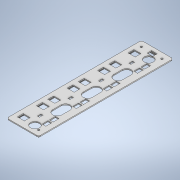
# Autodesk Inventor part: BoxLid
Saved by Autodesk Inventor 2021 (Build 250183000, 183)
## iProperties
Created: 2023-03-09
Part Number: BoxLid
Material: Generic
Document SubType Name: Modeling
Designer: mathe
Density: 1 g/cm^3
Appearance: Default
Author: mathe
Autodesk Inventor part; units mm, degrees
ref_plane "YZ Plane" through (0, 0, 0) normal (1, 0, 0) x (0, 1, 0)
ref_plane "XZ Plane" through (0, 0, 0) normal (0, 1, 0) x (-1, 0, 0)
ref_plane "XY Plane" through (0, 0, 0) normal (0, 0, 1) x (1, 0, 0)
sketch "Sketch1" plane through (0, 0, 0) normal (0, 1, 0) x (-1, 0, 0)
  line L0 (-9.707, 199.896) -> (-9.707, 209.896)
  line L1 (-9.707, 209.896) -> (2.293, 209.896)
  line L2 (2.293, 209.896) -> (2.293, 199.896)
  line L3 (2.293, 199.896) -> (-9.707, 199.896)
  line L4 (3.1921, 191.3679) -> (3.1921, 185.3679)
  line L5 (-9.707, 177.003) -> (2.293, 177.003)
  line L6 (-9.707, 167.003) -> (-9.707, 177.003)
  line L7 (2.293, 167.003) -> (-9.707, 167.003)
  line L8 (2.293, 177.003) -> (2.293, 167.003)
  line L9 (-9.707, 147.699) -> (-9.707, 157.699)
  line L10 (-9.707, 157.699) -> (2.293, 157.699)
  line L11 (2.293, 157.699) -> (2.293, 147.699)
  line L12 (2.293, 147.699) -> (-9.707, 147.699)
  line L13 (-9.707, 114.806) -> (-9.707, 124.806)
  line L14 (3.1921, 139.1709) -> (3.1921, 133.1709)
  line L15 (2.293, 124.806) -> (2.293, 114.806)
  line L16 (2.293, 114.806) -> (-9.707, 114.806)
  line L17 (-9.707, 124.806) -> (2.293, 124.806)
  circle A0 centre (-25.011, 102.489) radius 6.5
  circle A1 centre (-25.011, 116.713) radius 6.5
  line L18 (-9.707, 105.502) -> (2.293, 105.502)
  line L19 (2.293, 105.502) -> (2.293, 95.502)
  line L20 (2.293, 95.502) -> (-9.707, 95.502)
  line L21 (-9.707, 95.502) -> (-9.707, 105.502)
  line L22 (-17.0795, 87.0699) -> (-13.5395, 87.0699)
  line L23 (-35.859, 94.866) -> (-35.859, 84.866)
  circle A2 centre (-25.011, 12.319) radius 6.5
  line L24 (-9.707, 20.412) -> (2.293, 20.412)
  line L25 (2.293, 20.412) -> (2.293, 10.412)
  line L26 (2.293, 10.412) -> (-9.707, 10.412)
  line L27 (-9.707, 10.412) -> (-9.707, 20.412)
  line L28 (-17.686, -1.671) -> (-20.286, -1.671)
  circle A3 centre (-35.179, 0) radius 1.702
  line L29 (-20.461, 3.894) -> (-19.461, 3.894)
  line L30 (-23.811, 2.214) -> (-23.811, 0.214)
  line L31 (-14.161, 2.214) -> (-14.161, 0.214)
  circle A4 centre (0, 0) radius 1.702
  line L32 (-18.511, 3.894) -> (-17.511, 3.894)
  circle A5 centre (-25.011, 64.516) radius 6.5
  line L33 (-9.707, 72.609) -> (2.293, 72.609)
  line L34 (-9.707, 62.609) -> (-9.707, 72.609)
  line L35 (2.293, 62.609) -> (-9.707, 62.609)
  line L36 (2.293, 72.609) -> (2.293, 62.609)
  line L37 (3.1921, 86.9739) -> (3.1921, 80.9739)
  line L38 (-13.5395, 80.8699) -> (-17.0795, 80.8699)
  line L39 (-17.0795, 82.9738) -> (-17.0795, 84.9659)
  line L40 (-13.5395, 87.0699) -> (-13.5395, 80.8699)
  line L41 (-35.859, 82.293) -> (-35.859, 72.293)
  circle A6 centre (-25.011, 168.91) radius 6.5
  circle A7 centre (-25.011, 206.883) radius 6.5
  line L42 (-13.5395, 191.4639) -> (-13.5395, 185.2639)
  line L43 (-13.5395, 185.2639) -> (-17.0795, 185.2639)
  line L44 (-17.0795, 187.3678) -> (-17.0795, 189.3599)
  line L45 (-17.0795, 191.4639) -> (-13.5395, 191.4639)
  line L46 (-35.859, 186.687) -> (-35.859, 176.687)
  line L47 (-35.859, 199.26) -> (-35.859, 189.26)
  circle A8 centre (-35.179, 210.947) radius 1.702
  circle A9 centre (-25.011, 154.686) radius 6.5
  line L48 (-13.5395, 139.2668) -> (-13.5395, 133.0668)
  line L49 (-13.5395, 133.0668) -> (-17.0795, 133.0668)
  line L50 (-17.0795, 139.2668) -> (-13.5395, 139.2668)
  line L51 (-17.0795, 135.1708) -> (-17.0795, 137.1629)
  line L52 (-35.859, 134.49) -> (-35.859, 124.49)
  line L53 (-35.859, 147.063) -> (-35.859, 137.063)
  circle A10 centre (-25.011, 50.292) radius 6.5
  line L54 (-9.707, 53.305) -> (2.293, 53.305)
  line L55 (-9.707, 43.305) -> (-9.707, 53.305)
  line L56 (2.293, 43.305) -> (-9.707, 43.305)
  line L57 (2.293, 53.305) -> (2.293, 43.305)
  line L58 (3.1921, 34.7769) -> (3.1921, 28.7769)
  line L59 (-13.5395, 28.6728) -> (-17.0795, 28.6728)
  line L60 (-17.0795, 30.7768) -> (-17.0795, 32.7689)
  line L61 (-13.5395, 34.8728) -> (-13.5395, 28.6728)
  line L62 (-17.0795, 34.8728) -> (-13.5395, 34.8728)
  line L63 (-35.859, 30.096) -> (-35.859, 20.096)
  line L64 (-35.859, 42.669) -> (-35.859, 32.669)
  line L65 (9.525, 220.472) -> (-44.704, 220.472)
  line L66 (-44.704, 220.472) -> (-44.704, -9.525)
  line L67 (-44.704, -9.525) -> (9.525, -9.525)
  line L68 (9.525, -9.525) -> (9.525, 220.472)
  line L69 (6.35, -6.35) -> (-41.529, -6.35)
  line L70 (-41.529, -6.35) -> (-41.529, 217.297)
  line L71 (-41.529, 217.297) -> (6.35, 217.297)
  line L72 (6.35, 217.297) -> (6.35, -6.35)
  line L73 (-13.5395, 191.4639) -> (-17.0795, 191.4639)
  line L74 (-17.0795, 191.4639) -> (-17.0795, 185.2639)
  line L75 (-17.0795, 185.2639) -> (-13.5395, 185.2639)
  line L76 (-13.5395, 185.2639) -> (-13.5395, 191.4639)
  line L77 (-13.5395, 139.2668) -> (-17.0795, 139.2668)
  line L78 (-17.0795, 139.2668) -> (-17.0795, 133.0668)
  line L79 (-17.0795, 133.0668) -> (-13.5395, 133.0668)
  line L80 (-13.5395, 133.0668) -> (-13.5395, 139.2668)
  line L81 (-13.5395, 87.0699) -> (-17.0795, 87.0699)
  line L82 (-17.0795, 87.0699) -> (-17.0795, 80.8699)
  line L83 (-17.0795, 80.8699) -> (-13.5395, 80.8699)
  line L84 (-13.5395, 80.8699) -> (-13.5395, 87.0699)
  line L85 (-13.5395, 34.8728) -> (-17.0795, 34.8728)
  line L86 (-17.0795, 34.8728) -> (-17.0795, 28.6728)
  line L87 (-17.0795, 28.6728) -> (-13.5395, 28.6728)
  line L88 (-13.5395, 28.6728) -> (-13.5395, 34.8728)
  circle A11 centre (-25.011, 206.883) radius 7.77
  circle A12 centre (-25.011, 168.91) radius 7.77
  circle A13 centre (-25.011, 154.686) radius 7.77
  circle A14 centre (-25.011, 116.713) radius 7.77
  circle A15 centre (-25.011, 102.489) radius 7.77
  circle A16 centre (-25.011, 64.516) radius 7.77
  circle A17 centre (-25.011, 50.292) radius 7.77
  circle A18 centre (-25.011, 12.319) radius 7.77
  line L89 (-17.241, 168.91) -> (-32.781, 168.91)
  line L90 (-32.781, 168.91) -> (-32.781, 154.686)
  line L91 (-32.781, 154.686) -> (-17.241, 154.686)
  line L92 (-17.241, 154.686) -> (-17.241, 168.91)
  line L93 (-17.241, 116.713) -> (-32.781, 116.713)
  line L94 (-32.781, 116.713) -> (-32.781, 102.489)
  line L95 (-32.781, 102.489) -> (-17.241, 102.489)
  line L96 (-17.241, 102.489) -> (-17.241, 116.713)
  line L97 (-17.241, 64.516) -> (-32.781, 64.516)
  line L98 (-32.781, 64.516) -> (-32.781, 50.292)
  line L99 (-32.781, 50.292) -> (-17.241, 50.292)
  line L100 (-17.241, 50.292) -> (-17.241, 64.516)
  line L101 (-35.859, 199.26) -> (-29.509, 199.26)
  line L102 (-29.509, 199.26) -> (-29.509, 189.26)
  line L103 (-29.509, 189.26) -> (-35.859, 189.26)
  line L104 (-35.859, 189.26) -> (-35.859, 199.26)
  line L105 (-35.859, 186.687) -> (-29.509, 186.687)
  line L106 (-29.509, 186.687) -> (-29.509, 176.68)
  line L107 (-29.509, 176.68) -> (-35.859, 176.68)
  line L108 (-35.859, 176.68) -> (-35.859, 186.687)
  line L109 (-35.859, 147.063) -> (-29.509, 147.063)
  line L110 (-29.509, 147.063) -> (-29.509, 137.063)
  line L111 (-29.509, 137.063) -> (-35.859, 137.063)
  line L112 (-35.859, 137.063) -> (-35.859, 147.063)
  line L113 (-35.859, 134.49) -> (-29.509, 134.49)
  line L114 (-29.509, 134.49) -> (-29.509, 124.483)
  line L115 (-29.509, 124.483) -> (-35.859, 124.483)
  line L116 (-35.859, 124.483) -> (-35.859, 134.49)
  line L117 (-35.859, 94.866) -> (-29.509, 94.866)
  line L118 (-29.509, 94.866) -> (-29.509, 84.9659)
  line L119 (-29.509, 84.9659) -> (-35.859, 84.9659)
  line L120 (-35.859, 84.9659) -> (-35.859, 94.866)
  line L121 (-35.859, 82.293) -> (-29.509, 82.293)
  line L122 (-29.509, 82.293) -> (-29.509, 72.286)
  line L123 (-29.509, 72.286) -> (-35.859, 72.286)
  line L124 (-35.859, 72.286) -> (-35.859, 82.293)
  line L125 (-35.859, 42.522) -> (-29.509, 42.522)
  line L126 (-29.509, 42.522) -> (-29.509, 32.669)
  line L127 (-29.509, 32.669) -> (-35.859, 32.669)
  line L128 (-35.859, 32.669) -> (-35.859, 42.522)
  line L129 (-35.859, 30.096) -> (-29.509, 30.096)
  line L130 (-29.509, 30.096) -> (-29.509, 20.089)
  line L131 (-29.509, 20.089) -> (-35.859, 20.089)
  line L132 (-35.859, 20.089) -> (-35.859, 30.096)
  line L133 (-14.161, 3.894) -> (-23.811, 3.894)
  line L134 (-23.811, 3.894) -> (-23.811, -1.671)
  line L135 (-23.811, -1.671) -> (-14.161, -1.671)
  line L136 (-14.161, -1.671) -> (-14.161, 3.894)
  line L137 (-14.161, 3.894) -> (-23.811, 3.894)
  line L138 (-23.811, 3.894) -> (-23.811, -3.091)
  line L139 (-23.811, -3.091) -> (-14.161, -3.091)
  line L140 (-14.161, -3.091) -> (-14.161, 3.894)
  line L141 (-14.161, -1.671) -> (-23.811, -1.671)
  line L142 (-23.811, -1.671) -> (-23.811, 4.425)
  line L143 (-23.811, 4.425) -> (-14.161, 4.425)
  line L144 (-14.161, 4.425) -> (-14.161, -1.671)
  point P0 (0, 0)
  point P1 (0, 0)
  point P2 (-17.0795, 34.8728)
  point P3 (-17.0795, 87.0699)
  point P4 (-17.0795, 139.2668)
  point P5 (-17.0795, 191.4639)
  point P6 (-17.241, 50.292)
  point P7 (-17.241, 102.489)
  point P8 (-17.241, 154.686)
  point P9 (-35.859, 84.9659)
  point P10 (-23.811, 0.214)
  point P11 (-23.811, -1.671)
  point P12 (-14.161, 0.214)
  dimension "d0" = 1.27
  dimension "d1" = 1.27
  dimension "d2" = 1.27
  dimension "d3" = 1.27
  dimension "d4" = 1.27
  dimension "d5" = 1.27
  dimension "d6" = 1.27
  dimension "d7" = 1.27
  dimension "d12" = 6.35
  dimension "d16" = 6.985
  dimension "d17" = 6.096
  constraints: 290 end point, 36 parallel, 18 horizontal, 18 perpendicular, 13 centre point, 10 point on line, 18 other
  measures "d0" radial gap between concentric circles of A7 A11
  measures "d7" radial gap between concentric circles of A2 A18
  measures "d12" distance of L102.end L103.end
  measures "d16" distance of L138.end L137.end
  measures "d17" distance of L141.end L142.end
extrude "Extrusion1" add sketch "Sketch1" against normal blind 4.7625 contours L117 L118 L119 L23 | L135 L140 L139 L138 L28 | L28 L135 L134 L30 L133 L29 L32 L136 L31 | L133 L32 L29 L142 L143 L144 | L121 L122 L123 L124 L41 | L105 L106 L107 L108 L46 | L101 L102 L103 L47 | L113 L114 L115 L116 L52 | L109 L110 L111 L53 | L129 L130 L131 L132 L63 | L125 L126 L127 L64 | L69 L70 L71 L72
extrude "Extrusion2" add sketch "Sketch1" against normal blind 1.7145 contours L68 L67 L66 L65
extrude "Extrusion3" cut sketch "Sketch1" against normal up to surface (4.7625 mm away) contours L117 L118 L119 L23 | L135 L140 L139 L138 L28 | L28 L135 L134 L30 L133 L29 L32 L136 L31 | L133 L32 L29 L142 L143 L144 | L121 L122 L123 L124 L41 | L105 L106 L107 L108 L46 | L101 L102 L103 L47 | L113 L114 L115 L116 L52 | L109 L110 L111 L53 | L129 L130 L131 L132 L63 | L125 L126 L127 L64
fillet "Fillet1" radius 3.175 4 edges at (44.704, -0.8573, -9.525) (-9.525, -0.8573, -9.525) (-9.525, -0.8573, 220.472) (44.704, -0.8573, 220.472)
sketch "Sketch2" plane through (0, -4.7625, 0) normal (0, -1, 0) x (1, 0, 0)
  line L0 (29.509, 176.68) -> (29.509, 186.687) projected
  line L1 (29.509, 186.687) -> (35.859, 186.687) projected
  line L2 (35.859, 186.687) -> (35.859, 176.68) projected
  line L3 (35.859, 176.68) -> (29.509, 176.68) projected
  line L4 (14.161, -3.091) -> (14.161, 4.425) projected
  line L5 (14.161, 4.425) -> (23.811, 4.425) projected
  line L6 (23.811, 4.425) -> (23.811, -3.091) projected
  line L7 (23.811, -3.091) -> (14.161, -3.091) projected
  line L8 (35.859, 124.483) -> (29.509, 124.483) projected
  line L9 (29.509, 124.483) -> (29.509, 134.49) projected
  line L10 (29.509, 134.49) -> (35.859, 134.49) projected
  line L11 (35.859, 134.49) -> (35.859, 124.483) projected
  line L12 (29.509, 20.089) -> (29.509, 30.096) projected
  line L13 (29.509, 30.096) -> (35.859, 30.096) projected
  line L14 (35.859, 30.096) -> (35.859, 20.089) projected
  line L15 (35.859, 20.089) -> (29.509, 20.089) projected
  line L16 (29.509, 84.9659) -> (29.509, 94.866) projected
  line L17 (29.509, 94.866) -> (35.859, 94.866) projected
  line L18 (35.859, 94.866) -> (35.859, 84.9659) projected
  line L19 (35.859, 84.9659) -> (29.509, 84.9659) projected
  line L20 (29.509, 189.26) -> (29.509, 199.26) projected
  line L21 (29.509, 199.26) -> (35.859, 199.26) projected
  line L22 (35.859, 199.26) -> (35.859, 189.26) projected
  line L23 (35.859, 189.26) -> (29.509, 189.26) projected
  line L24 (35.859, 137.063) -> (29.509, 137.063) projected
  line L25 (29.509, 137.063) -> (29.509, 147.063) projected
  line L26 (29.509, 147.063) -> (35.859, 147.063) projected
  line L27 (35.859, 147.063) -> (35.859, 137.063) projected
  line L28 (29.509, 32.669) -> (29.509, 42.522) projected
  line L29 (29.509, 42.522) -> (35.859, 42.522) projected
  line L30 (35.859, 42.522) -> (35.859, 32.669) projected
  line L31 (35.859, 32.669) -> (29.509, 32.669) projected
  line L32 (35.859, 72.286) -> (29.509, 72.286) projected
  line L33 (29.509, 72.286) -> (29.509, 82.293) projected
  line L34 (29.509, 82.293) -> (35.859, 82.293) projected
  line L35 (35.859, 82.293) -> (35.859, 72.286) projected
  line L36 (41.529, -6.35) -> (41.529, 217.297) projected
  line L37 (41.529, 217.297) -> (-6.35, 217.297) projected
  line L38 (-6.35, 217.297) -> (-6.35, -6.35) projected
  line L39 (-6.35, -6.35) -> (41.529, -6.35) projected
  line L40 (17.0795, 34.8728) -> (17.0795, 28.6728) projected
  line L41 (17.0795, 28.6728) -> (13.5395, 28.6728) projected
  line L42 (13.5395, 28.6728) -> (13.5395, 34.8728) projected
  line L43 (13.5395, 34.8728) -> (17.0795, 34.8728) projected
  circle A0 centre (35.179, 210.947) radius 1.702 projected
  circle A1 centre (0, 0) radius 1.702 projected
  line L44 (17.0795, 87.0699) -> (17.0795, 80.8699) projected
  line L45 (17.0795, 80.8699) -> (13.5395, 80.8699) projected
  line L46 (13.5395, 80.8699) -> (13.5395, 87.0699) projected
  line L47 (13.5395, 87.0699) -> (17.0795, 87.0699) projected
  circle A2 centre (35.179, 0) radius 1.702 projected
  line L48 (17.0795, 139.2668) -> (17.0795, 133.0668) projected
  line L49 (17.0795, 133.0668) -> (13.5395, 133.0668) projected
  line L50 (13.5395, 133.0668) -> (13.5395, 139.2668) projected
  line L51 (13.5395, 139.2668) -> (17.0795, 139.2668) projected
  line L52 (17.0795, 191.4639) -> (17.0795, 185.2639) projected
  line L53 (17.0795, 185.2639) -> (13.5395, 185.2639) projected
  line L54 (13.5395, 185.2639) -> (13.5395, 191.4639) projected
  line L55 (13.5395, 191.4639) -> (17.0795, 191.4639) projected
  circle A3 centre (25.011, 12.319) radius 7.77 projected
  circle A4 centre (25.011, 206.883) radius 7.77 projected
  line L56 (-2.293, 53.305) -> (9.707, 53.305) projected
  line L57 (9.707, 53.305) -> (9.707, 43.305) projected
  line L58 (9.707, 43.305) -> (-2.293, 43.305) projected
  line L59 (-2.293, 43.305) -> (-2.293, 53.305) projected
  line L60 (-2.293, 72.609) -> (9.707, 72.609) projected
  line L61 (9.707, 72.609) -> (9.707, 62.609) projected
  line L62 (9.707, 62.609) -> (-2.293, 62.609) projected
  line L63 (-2.293, 62.609) -> (-2.293, 72.609) projected
  line L64 (-2.293, 20.412) -> (9.707, 20.412) projected
  line L65 (9.707, 20.412) -> (9.707, 10.412) projected
  line L66 (9.707, 10.412) -> (-2.293, 10.412) projected
  line L67 (-2.293, 10.412) -> (-2.293, 20.412) projected
  line L68 (9.707, 147.699) -> (-2.293, 147.699) projected
  line L69 (-2.293, 147.699) -> (-2.293, 157.699) projected
  line L70 (-2.293, 157.699) -> (9.707, 157.699) projected
  line L71 (9.707, 157.699) -> (9.707, 147.699) projected
  line L72 (-2.293, 105.502) -> (9.707, 105.502) projected
  line L73 (9.707, 105.502) -> (9.707, 95.502) projected
  line L74 (9.707, 95.502) -> (-2.293, 95.502) projected
  line L75 (-2.293, 95.502) -> (-2.293, 105.502) projected
  line L76 (-2.293, 124.806) -> (9.707, 124.806) projected
  line L77 (9.707, 124.806) -> (9.707, 114.806) projected
  line L78 (9.707, 114.806) -> (-2.293, 114.806) projected
  line L79 (-2.293, 114.806) -> (-2.293, 124.806) projected
  line L80 (9.707, 167.003) -> (-2.293, 167.003) projected
  line L81 (-2.293, 167.003) -> (-2.293, 177.003) projected
  line L82 (-2.293, 177.003) -> (9.707, 177.003) projected
  line L83 (9.707, 177.003) -> (9.707, 167.003) projected
  line L84 (9.707, 209.896) -> (9.707, 199.896) projected
  line L85 (9.707, 199.896) -> (-2.293, 199.896) projected
  line L86 (-2.293, 199.896) -> (-2.293, 209.896) projected
  line L87 (-2.293, 209.896) -> (9.707, 209.896) projected
  line L88 (17.241, 50.292) -> (17.241, 64.516) projected
  arc A5 (32.781, 64.516) -> (17.241, 64.516) centre (25.011, 64.516) ccw projected
  line L89 (32.781, 64.516) -> (32.781, 50.292) projected
  arc A6 (17.241, 50.292) -> (32.781, 50.292) centre (25.011, 50.292) ccw projected
  line L90 (17.241, 102.489) -> (17.241, 116.713) projected
  arc A7 (32.781, 116.713) -> (17.241, 116.713) centre (25.011, 116.713) ccw projected
  line L91 (32.781, 116.713) -> (32.781, 102.489) projected
  arc A8 (17.241, 102.489) -> (32.781, 102.489) centre (25.011, 102.489) ccw projected
  line L92 (17.241, 154.686) -> (17.241, 168.91) projected
  arc A9 (32.781, 168.91) -> (17.241, 168.91) centre (25.011, 168.91) ccw projected
  line L93 (32.781, 168.91) -> (32.781, 154.686) projected
  arc A10 (17.241, 154.686) -> (32.781, 154.686) centre (25.011, 154.686) ccw projected
  line L94 (-3.81, -3.81) -> (-3.81, 214.757)
  line L95 (-3.81, 214.757) -> (38.989, 214.757)
  line L96 (38.989, 214.757) -> (38.989, -3.81)
  line L97 (38.989, -3.81) -> (-3.81, -3.81)
  point P0 (0, 0)
  dimension "d19" = 2.54
  constraints: 8 end point, 3 other
  measures "d19" distance between parallel lines of L38 L94
extrude "Extrusion4" cut sketch "Sketch2" against normal up to surface (3.048 mm away) contours L94 L95 L96 L97
body "Solid1"
